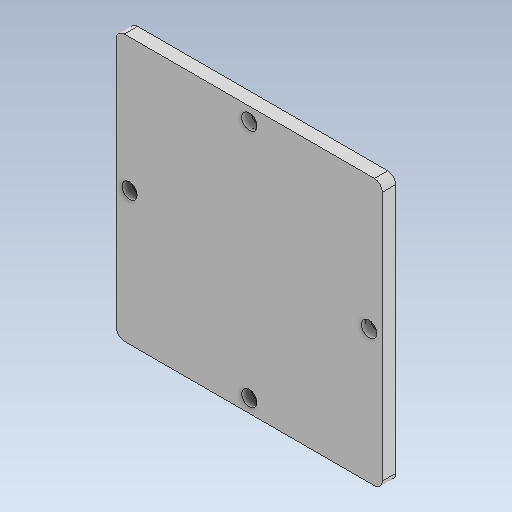
# Autodesk Inventor part: BaseBottom
Saved by Autodesk Inventor 2020 (Build 240168000, 168)
## iProperties
Created: 2020-08-08
Part Number: BaseBottom
Material: Generic
Document SubType Name: Modeling
Designer: reide
Density: 1 g/cm^3
Appearance: Default
Author: reide
Autodesk Inventor part; units mm, degrees
ref_plane "YZ Plane" through (0, 0, 0) normal (1, 0, 0) x (0, 1, 0)
ref_plane "XZ Plane" through (0, 0, 0) normal (0, 1, 0) x (-1, 0, 0)
ref_plane "XY Plane" through (0, 0, 0) normal (0, 0, 1) x (1, 0, 0)
sketch "Sketch1" plane through (0, 0, 0) normal (0, 0, 1) x (1, 0, 0)
  line L0 (47, 50) -> (-47, 50) projected
  line L1 (-50, 47) -> (-50, -47) projected
  line L2 (-47, -50) -> (47, -50) projected
  line L3 (50, -47) -> (50, 47) projected
  line L4 (-48, 4) -> (-48, 48) projected
  line L5 (4, 48) -> (48, 48) projected
  line L6 (48, 48) -> (48, 4) projected
  line L7 (48, -48) -> (4, -48) projected
  arc A0 (47, -50) -> (50, -47) centre (47, -47) ccw projected
  arc A1 (50, 47) -> (47, 50) centre (47, 47) ccw projected
  arc A2 (-47, 50) -> (-50, 47) centre (-47, 47) ccw projected
  arc A3 (-50, -47) -> (-47, -50) centre (-47, -47) ccw projected
  circle A4 centre (0, -45) radius 1.25 projected
  circle A5 centre (0, 45) radius 1.25 projected
  circle A6 centre (-45, 0) radius 1.25 projected
  circle A7 centre (45, 0) radius 1.25 projected
  arc A8 (-43, -3) -> (-42, -2) centre (-43, -2) ccw projected
  line L8 (-42, -2) -> (-42, 2) projected
  arc A9 (-42, 2) -> (-43, 3) centre (-43, 2) ccw projected
  line L9 (-43, 3) -> (-47, 3) projected
  arc A10 (-48, 4) -> (-47, 3) centre (-47, 4) ccw projected
  arc A11 (-3, 47) -> (-4, 48) centre (-4, 47) ccw projected
  line L10 (-3, 47) -> (-3, 43) projected
  arc A12 (-3, 43) -> (-2, 42) centre (-2, 43) ccw projected
  line L11 (-2, 42) -> (2, 42) projected
  arc A13 (2, 42) -> (3, 43) centre (2, 43) ccw projected
  line L12 (3, 43) -> (3, 47) projected
  arc A14 (4, 48) -> (3, 47) centre (4, 47) ccw projected
  arc A15 (47, 3) -> (48, 4) centre (47, 4) ccw projected
  line L13 (47, 3) -> (43, 3) projected
  arc A16 (43, 3) -> (42, 2) centre (43, 2) ccw projected
  line L14 (42, 2) -> (42, -2) projected
  arc A17 (42, -2) -> (43, -3) centre (43, -2) ccw projected
  line L15 (43, -3) -> (47, -3) projected
  arc A18 (48, -4) -> (47, -3) centre (47, -4) ccw projected
  arc A19 (3, -47) -> (4, -48) centre (4, -47) ccw projected
  line L16 (3, -47) -> (3, -43) projected
  arc A20 (3, -43) -> (2, -42) centre (2, -43) ccw projected
  line L17 (2, -42) -> (-2, -42) projected
  arc A21 (-2, -42) -> (-3, -43) centre (-2, -43) ccw projected
  line L18 (-3, -43) -> (-3, -47) projected
  arc A22 (-4, -48) -> (-3, -47) centre (-4, -47) ccw projected
  arc A23 (-47, -3) -> (-48, -4) centre (-47, -4) ccw projected
  line L19 (-47, -3) -> (-43, -3) projected
  line L20 (-48, 48) -> (-4, 48) projected
  line L21 (48, -4) -> (48, -48) projected
  line L22 (-4, -48) -> (-48, -48) projected
  line L23 (-48, -48) -> (-48, -4) projected
  point P0 (0, 0)
  point P1 (-47, 4)
  point P2 (-4, 47)
  point P3 (4, 47)
  point P4 (47, 4)
  point P5 (47, -4)
  point P6 (4, -47)
  point P7 (-4, -47)
  point P8 (-47, -4)
extrude "Extrusion1" add sketch "Sketch1" along normal blind 5 contours A1 L3 A0 L2 A3 L1 A2 L0 | L4 L20 A11 L10 A12 L11 A13 L12 A14 L5 L6 A15 L13 A16 L14 A17 L15 A18 L21 L7 A19 L16 A20 L17 A21 L18 A22 L22 L23 A23 L19 A8 L8 A9 L9 A10
sketch "Sketch2" plane through (0, 0, 5) normal (0, 0, 1) x (1, 0, 0)
  circle A0 centre (45, 0) radius 1.25 projected
  circle A1 centre (45, 0) radius 2.875
  circle A2 centre (0, 45) radius 2.875
  circle A3 centre (-45, 0) radius 2.875
  circle A4 centre (0, -45) radius 2.875
  point P0 (0, 0)
  dimension "d2" = 5.75
  dimension "d5" = 360
  constraints: 4 centre point, 1 coincident, 9 other
  measures "d2" diameter of A1
extrude "Extrusion2" cut sketch "Sketch2" against normal blind 3.5 contours A0 | A1 | A2 | A3 | A4
sketch "Sketch3" plane through (0, 0, 0) normal (0, 0, -1) x (-1, 0, 0)
  line L0 (-42, 42) -> (42, 42)
  line L1 (42, 42) -> (42, -42)
  line L2 (42, -42) -> (-42, -42)
  line L3 (-42, -42) -> (-42, 42)
  line L4 (-42, 42) -> (42, -42) construction
  line L5 (42, 42) -> (-42, -42) construction
  point P0 (0, 0)
  dimension "d9" = 84
  dimension "d10" = 84
  constraints: 12 end point, 2 midpoint, 2 parallel, 1 horizontal, 1 perpendicular
  measures "d9" distance of L0.start L0.end
  measures "d10" distance of L0.end L1.end
extrude "Extrusion3" cut sketch "Sketch3" against normal blind 3.5
body "Solid1"
